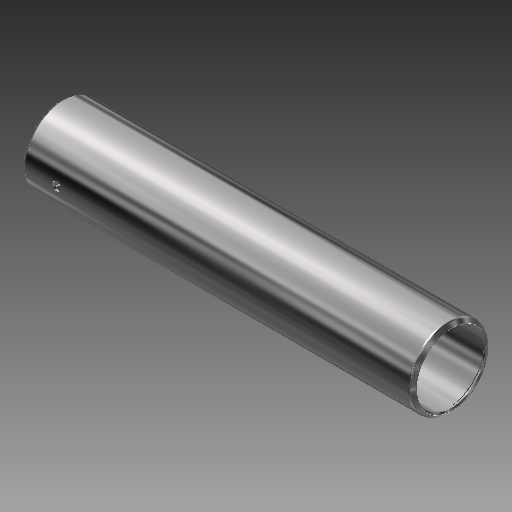
# Autodesk Inventor part: 04-3.9452C
Saved by Autodesk Inventor 2017 (Build 210142000, 142)
## iProperties
Category: PARTsolutions
Company: BIMBA
Created: 2016-10-01
Part Number: 04-3.9452C
Catalog Web Link: www.cadenas.de
Description: Tube-Original Line - Standard Air Cylinders
Vendor: BIMBA
Document SubType Name: Modeling
Designer: psAdmin
Manufacturer: BIMBA
Mass: 28.3203 g
Surface Area: 127.79 cm^2
Volume: 3.54004 cm^3
Density: 8 g/cm^3
Material: Stainless Steel
Appearance: Semi-Polished
PSOL_IDENT_0: {$CADENAS_DATA\23d-libs\bimba\bimba\bimba_imperial\bimba_full_line\original_line_cylinders\standard_
PSOL_IDENT_1: air_cylinders\tube.prj},188 {VTYP=3D},{NB=04-3.9452C},{LINA=04-3.9452C},{NN=Tube},{DATE=22.09.2016 1
PSOL_IDENT_2: 3:52:25},{GEOMDATE=18.02.2011 00:00:00},{VERSION=},{LINEID=40},{LINESUBID=-1},{WBVAR=MNT,ACTING,NR,L
PSOL_IDENT_3: ,FOURHOLES,SR}  {NB=04-3.9452C},{LINA=04-3.9452C},{KT=DUMMY},{PN=04-3.9452C},{BORE=0.75000000},{BORE
PSOL_IDENT_4: PN=04},{MNT=},{MNTALG='' , 'Front Nose' , 'BF' , 'Front Block' , 'BFT' , 'Front Trunnion' , 'A' , 'A
PSOL_IDENT_5: djustable Stroke'},{ACTING=},{ACTINGALG= '' , 'Single Acting' , 'R' , 'Reverse/Double Acting' },{NR=
PSOL_IDENT_6: },{NRALG= '' , 'Without Non-rotating Rod' , 'NR' , 'With Non-rotating Rod' },{L=3.9450},{OD=0.8050},
PSOL_IDENT_7: {ODN=0.8050},{ODP=0.8625},{ODB=0.8325},{ID=0.7615},{DV=0.00000000},{LV=0.00000000},{LV1=0.00000000},
PSOL_IDENT_8: {G=0.0300},{FOURHOLES=2},{AA=0.3750},{BB=0.0940},{SR=C},{SRALG= 'C' , 'Carbon Steel Rod' , 'SR' , '3
PSOL_IDENT_9: 03 Stainless Steel Rod' , '' , '303 Stainless Steel Rod'}
NN: Tube
NT: Original Line - Standard Air Cylinders
NB: 04-3.9452C
NBSYN: $PN.
LINA: 04-3.9452C
BORE: 3/4
BOREPN: 04
MNT: Front Nose
MNTALG: '' , 'Front Nose' , 'BF' , 'Front Block' , 'BFT' , 'Front Trunnion' , 'A' , 'Adjustable Stroke'
ACTING: Single Acting
NR: Without Non-rotating Rod
L: 3.9450
ODN: 0.8050
ODP: 0.8625
ODB: 0.8325
ID: 0.7615
DV: 0.00000000
LV: 0.00000000
LV1: 0.00000000
G: 0.0300
FOURHOLES: 2
AA: 0.3750
BB: 0.0940
SR: Carbon Steel Rod
SUPPLIER: BIMBA
ARTICLENO: 04-3.9452C
BOMINFO: 04-3.9452C
CREATOR: CADENAS GmbH
Title: 04-3.9452C
Author: Cadenas PARTsolutions
Comments: Original Line - Standard Air Cylinders
Autodesk Inventor part; units mm, degrees
sketch "Sketch_1" plane through (0, 0, 0) normal (0, 0, 1) x (1, 0, 0)
  line L0 (100.203, 0) -> (0, 0)
  arc A0 (-0.6395, 9.3472) -> (-0.6395, 9.1676) centre (-0.5497, 9.2574) ccw
  line L1 (-0.6395, 9.1676) -> (-0.381, 8.9091)
  line L2 (-0.381, 8.9091) -> (0, 8.9091)
  line L3 (0, 8.9091) -> (0.762, 9.671)
  line L4 (0.762, 9.671) -> (99.441, 9.671)
  line L5 (99.441, 9.671) -> (100.203, 8.9091)
  line L6 (100.203, 8.9091) -> (100.584, 8.9091)
  line L7 (100.584, 8.9091) -> (100.8425, 9.1676)
  arc A1 (100.8425, 9.1676) -> (100.8425, 9.3472) centre (100.7527, 9.2574) ccw
  line L8 (100.8425, 9.3472) -> (100.1894, 10.0003)
  arc A2 (100.1894, 10.0003) -> (99.6505, 10.2235) centre (99.6506, 9.4615) ccw
  line L9 (99.6505, 10.2235) -> (0.5524, 10.2235)
  arc A3 (0.5524, 10.2235) -> (0.0136, 10.0003) centre (0.5524, 9.4615) ccw
  line L10 (0.0136, 10.0003) -> (-0.6395, 9.3472)
  constraints: 22 end point, 8 point on circle, 4 centre point
revolve "Revolution1" add sketch "Sketch_1" angle 360 about axis through (100.203, 0, 0) along (1, 0, 0)
sketch "Sketch_4" plane through (0, 0, 0) normal (0, 0, 1) x (1, 0, 0)
  circle A0 centre (8.763, 0) radius 1.1938
  constraints: 1 centre point
extrude "Extrusion1" cut sketch "Sketch_4" along normal blind 10.2235
ref_plane "cp1_XY" through (50.1015, 10.2235, 0) normal (1, 0, 0) x (0, 0, -1)
ref_plane "cp1_YZ" through (50.1015, 10.2235, 0) normal (0, 0, -1) x (0, 1, 0)
ref_plane "cp1_ZX" through (50.1015, 10.2235, 0) normal (0, 1, 0) x (1, 0, 0)
ref_plane "cp2_XY" through (50.1015, 0, -10.2235) normal (1, 0, 0) x (0, 0, -1)
ref_plane "cp2_YZ" through (50.1015, 0, -10.2235) normal (0, 0, -1) x (0, 1, 0)
ref_plane "cp2_ZX" through (50.1015, 0, -10.2235) normal (0, 1, 0) x (1, 0, 0)
ref_plane "cp3_XY" through (50.1015, -10.2235, 0) normal (1, 0, 0) x (0, 0, -1)
ref_plane "cp3_YZ" through (50.1015, -10.2235, 0) normal (0, 0, -1) x (0, 1, 0)
ref_plane "cp3_ZX" through (50.1015, -10.2235, 0) normal (0, 1, 0) x (1, 0, 0)
ref_plane "cp4_XY" through (50.1015, 0, 10.2235) normal (1, 0, 0) x (0, 0, -1)
ref_plane "cp4_YZ" through (50.1015, 0, 10.2235) normal (0, 0, -1) x (0, 1, 0)
ref_plane "cp4_ZX" through (50.1015, 0, 10.2235) normal (0, 1, 0) x (1, 0, 0)
ref_plane "tube_front_XY" through (0, 0, 0) normal (1, 0, 0) x (0, 0, -1)
ref_plane "tube_front_YZ" through (0, 0, 0) normal (0, 0, -1) x (0, 1, 0)
ref_plane "tube_front_ZX" through (0, 0, 0) normal (0, 1, 0) x (1, 0, 0)
ref_plane "tube_rear_XY" through (100.203, 0, 0) normal (1, 0, 0) x (0, 0, -1)
ref_plane "tube_rear_YZ" through (100.203, 0, 0) normal (0, 0, -1) x (0, 1, 0)
ref_plane "tube_rear_ZX" through (100.203, 0, 0) normal (0, 1, 0) x (1, 0, 0)
body "Solid1"
